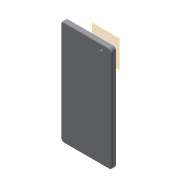
# Autodesk Inventor part: 100_Huawei_P9
Saved by Autodesk Inventor 2019 (Build 230136000, 136)
## iProperties
Created: 2019-05-31
Part Number: 100_Huawei_P9
Material: Generic
Document SubType Name: Modeling
Designer: diederichbenedict
Density: 1 g/cm^3
Appearance: Default
Author: diederichbenedict
Autodesk Inventor part; units mm, degrees
ref_plane "YZ Plane" through (0, 0, 0) normal (1, 0, 0) x (0, 1, 0)
ref_plane "XZ Plane" through (0, 0, 0) normal (0, 1, 0) x (-1, 0, 0)
ref_plane "XY Plane" through (0, 0, 0) normal (0, 0, 1) x (1, 0, 0)
ref_plane "Work Plane1" through (0, 0, 24.8) normal (0, 0, 1) x (1, 0, 0)
sketch "Sketch1" plane through (0, 0, 24.8) normal (0, 0, 1) x (1, 0, 0)
  circle A0 centre (0, 0) radius 2.1512
  line L0 (10.2, 7.3) -> (-50.7, 7.3)
  line L1 (-55.7, 2.3) -> (-55.7, -132.8)
  line L2 (-50.7, -137.8) -> (10.2, -137.8)
  line L3 (15.2, -132.8) -> (15.2, 2.3)
  arc A1 (-50.7, 7.3) -> (-55.7, 2.3) centre (-50.7, 2.3) ccw
  arc A2 (10.2, -137.8) -> (15.2, -132.8) centre (10.2, -132.8) ccw
  arc A3 (-55.7, -132.8) -> (-50.7, -137.8) centre (-50.7, -132.8) ccw
  arc A4 (15.2, 2.3) -> (10.2, 7.3) centre (10.2, 2.3) ccw
  point P0 (-55.7, -137.8)
  point P1 (-55.7, 7.3)
  point P2 (15.2, -137.8)
  dimension "d0" = 70.9
  dimension "d1" = 145.1
  dimension "d2" = 15.2
  dimension "d3" = 7.3
  dimension "d5" = 5
  constraints: 8 end point, 8 point on circle, 8 tangent, 6 point on line, 5 centre point, 3 equal radius, 2 parallel, 1 coincident, 1 horizontal, 1 perpendicular
  measures "d0" distance of point (15.2, -137.8) point (-55.7, -137.8)
  measures "d1" distance of point (-55.7, -137.8) point (-55.7, 7.3)
  measures "d2" distance from line of point (0, 0) L3
  measures "d3" distance from line of L0 point (0, 0)
  measures "d5" radius of A1
extrude "Extrusion1" add sketch "Sketch1" along normal blind 7.1
fillet "Fillet1" radius 2 16 edges at (13.7355, 5.8355, 31.9) (-20.25, 7.3, 31.9) (-54.2355, 5.8355, 31.9) (-55.7, -65.25, 31.9) (-54.2355, -136.3355, 31.9) (-20.25, -137.8, 31.9) (13.7355, -136.3355, 31.9) (15.2, -65.25, 31.9) (-54.2355, 5.8355, 24.8) (-55.7, -65.25, 24.8) (-54.2355, -136.3355, 24.8) (-20.25, -137.8, 24.8) (13.7355, -136.3355, 24.8) (15.2, -65.25, 24.8) (13.7355, 5.8355, 24.8) (-20.25, 7.3, 24.8)
body "Solid1"
